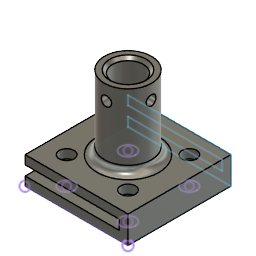
base_camara (Autodesk Fusion 360 design; units mm, degrees)
Autodesk Fusion 360 part; units mm, degrees
note: some values were not read from the file. Set by a fixed rule: which sketch regions a step uses.
sketch "Boceto1" plane through (0, 0, 0) normal (0, 0, 1) x (1, 0, 0)
  line L0 (-7, 15) -> (25, 15)
  line L1 (25, 15) -> (25, 11.7)
  line L2 (25, 11.7) -> (-7, 11.7)
  line L3 (-7, 11.7) -> (-7, 8.7)
  line L4 (-7, 8.7) -> (28, 8.7)
  line L5 (28, 8.7) -> (28, 18)
  line L6 (28, 18) -> (-7, 18)
  line L7 (-7, 18) -> (-7, 15)
  dimension "d1" = 3.3
  dimension "d2" = 3
  dimension "d3" = 3
  dimension "d4" = 3
  dimension "d5" = 35
  dimension "d6" = 35
  constraint horizontal L0
  constraint perpendicular L0 L1
  constraint perpendicular L1 L2
  constraint perpendicular L2 L3
  constraint perpendicular L3 L4
  constraint perpendicular L4 L5
  constraint perpendicular L3 L6
  constraint perpendicular L0 L7
  measures "d1" distance of L0 L2
  measures "d2" distance of L1 L5
  measures "d3" distance of L0 L6
  measures "d4" distance of L2 L4
  measures "d5" distance of L5 L7
  measures "d6" distance of L3 L5
extrude "Extruir1" add sketch "Boceto1" along normal blind 35
sketch "Boceto2" plane through (0, 18, 0) normal (0, 1, 0) x (-1, 0, 0)
  line L0 (-28, 35) -> (7, 0) construction
  line L1 (7, 35) -> (-28, 0) construction
  circle A0 centre (-10.5, 17.5) radius 8
  circle A1 centre (-10.5, 17.5) radius 5.2
  dimension "d35" = 16
  dimension "d60" = 10.4
  constraint midpoint L1 A0.centre
  constraint concentric A0 A1
  measures "d35" diameter of A0
  measures "d60" diameter of A1
extrude "Extruir4" add sketch "Boceto2" along normal blind 25
sketch "Boceto4" plane through (0, 18, 0) normal (0, 1, 0) x (-1, 0, 0)
  circle A0 centre (-10.5, 17.5) radius 8
  line L0 (7, 35) -> (-4.8431, 23.1569)
  line L1 (-16.1569, 11.8431) -> (-28, 0)
  line L2 (-28, 35) -> (-16.1569, 23.1569) construction
  line L3 (-4.8431, 11.8431) -> (7, 0) construction
  circle A1 centre (-20.9289, 27.9289) radius 2.5
  line L4 (-10.5, 17.5) -> (-10.5, 29) construction
  line L5 (-10.5, 17.5) -> (1, 17.5) construction
  circle A2 centre (-0.0711, 27.9289) radius 2.5
  circle A3 centre (-0.0711, 7.0711) radius 2.5
  circle A4 centre (-20.9289, 7.0711) radius 2.5
  point P0 (-28, 35)
  dimension "d37" = 5
  dimension "d38" = 10
  constraint coincident A0 L0.end
  constraint collinear L0 L1
  constraint coincident A0 L1.start
  constraint coincident A0 L2.end
  constraint coincident A0 L3.start
  constraint collinear L2 L3
  constraint coincident L2 A1.centre
  constraint coincident A0.centre L4.start
  constraint vertical L4
  constraint perpendicular L4 L5
  constraint symmetric A1 L4 A2
  constraint symmetric A1 L5 A4
  constraint symmetric L5 A2 A3
  measures "d37" diameter of A1
  measures "d38" distance of A1.centre P0
extrude "Extruir7" cut sketch "Boceto4" against normal through all contours L0 A2 | L0 A2 | L1 A4 | L1 A4 | A1 | A3
ref_plane "PlanoDeObra1" through (2.5, 43, 17.5) normal (0, 0, 1) x (1, 0, 0)
sketch "Boceto7" plane through (2.5, 43, 17.5) normal (0, 0, 1) x (1, 0, 0)
ref_plane "PlanoDeObra2" through (10.5, 35.1585, 25.5) normal (0, 0, 1) x (-1, 0, 0)
sketch "Boceto8" plane through (0, 0, 25.5) normal (0, 0, 1) x (1, 0, 0)
  line L0 (11, 50.5) -> (11, 25.5) construction
  circle A0 centre (11, 38) radius 1.65
  line L1 (28, 18) -> (-7, 18)
  dimension "d58" = 3.3
  dimension "d59" = 20
  constraint midpoint L0 A0.centre
  measures "d58" diameter of A0
  measures "d59" distance of A0.centre L1
extrude "Extruir9" cut sketch "Boceto8" along normal up to surface end surface at (5.3258, 26.3333, 16.9822)
ref_plane "PlanoDeObra3" through (10.5, 0, 0) normal (1, 0, 0) x (0, 1, 0)
sketch "Boceto9" plane through (10.5, 0, 0) normal (1, 0, 0) x (0, 0, -1)
  circle A0 centre (-17.5, 38) radius 1.65
  point P0 (-17.5, 18)
  dimension "d51" = 3.3
  dimension "d52" = 20
  measures "d51" diameter of A0
  measures "d52" distance of A0.centre P0
extrude "Extruir10" cut sketch "Boceto9" along normal through all
fillet "Empalme1" radius 2.5 1 edges at (17.9586, 18, 20.3929)
chamfer "Chaflán1" distance 1 angle 45 1 edges at (15.3481, 43, 19.3804)
sketch "Boceto11" plane through (0, 8.7, 0) normal (0, -1, 0) x (1, 0, 0)
  circle A0 centre (20.9289, 7.0711) radius 2.5
  circle A1 centre (0.0711, 27.9289) radius 2.5
  circle A2 centre (20.9289, 27.9289) radius 2.5
  circle A3 centre (0.0711, 7.0711) radius 2.5
  line L0 (-7, 0) -> (28, 0)
  line L1 (28, 0) -> (28, 35)
  line L2 (28, 35) -> (-7, 35)
  line L3 (-7, 35) -> (-7, 0)
  line L4 (-7, 35) -> (28, 35)
  circle A4 centre (0.0711, 27.9289) radius 2.5
  circle A5 centre (20.9289, 27.9289) radius 2.5
  circle A6 centre (20.9289, 7.0711) radius 2.5
  circle A7 centre (0.0711, 7.0711) radius 2.5
  dimension "d61" = 20.8579
  dimension "d62" = 20.8579
  dimension "d63" = 7.0711
  measures "d61" distance of A2.centre A1.centre
  measures "d62" distance of A3.centre A1.centre
  measures "d63" distance of A1.centre L2
